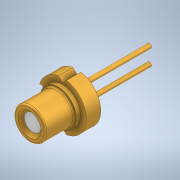
# Autodesk Inventor part: CAN_φ3.3
Saved by Autodesk Inventor 2020 (Build 240168000, 168)
## iProperties
Created: 2020-03-16
Part Number: CAN_φ3.3
Material: 黄铜，软黄
Document SubType Name: Modeling
Designer: John
Mass: 0.447561 g
Surface Area: 1.18166 cm^2
Volume: 0.0528407 cm^3
Density: 8.47 g/cm^3
Appearance: 黄铜 - 缎光
Author: John
Autodesk Inventor part; units mm, degrees
ref_plane "YZ Plane" through (0, 0, 0) normal (1, 0, 0) x (0, 1, 0)
ref_plane "XZ Plane" through (0, 0, 0) normal (0, 1, 0) x (-1, 0, 0)
ref_plane "XY Plane" through (0, 0, 0) normal (0, 0, 1) x (1, 0, 0)
sketch "草图1" plane through (0, 0, 0) normal (0, 0, 1) x (1, 0, 0)
  circle A0 centre (0, 0) radius 1.65
  circle A1 centre (0, 0) radius 0.55 construction
  line L0 (0, 1.65) -> (0, 1.35)
  line L1 (0, 1.35) -> (0.2766, 1.6266)
  line L2 (0, 1.35) -> (-0.2766, 1.6266)
  line L3 (0, 1.35) -> (0.3912, 1.35) construction
  line L4 (0, 0) -> (0, 1.65) construction
  line L5 (0, 0) -> (-1.65, 0) construction
  line L6 (0, 0) -> (0, -1.65) construction
  circle A2 centre (0, 0.55) radius 0.15
  circle A3 centre (0, -0.55) radius 0.15
  circle A4 centre (-0.55, 0) radius 0.15
  circle A5 centre (-0.55, 0) radius 0.4
  line L7 (0, -1.65) -> (0, -1.35)
  line L8 (0, -1.35) -> (0.2766, -1.6266)
  line L9 (0, -1.35) -> (-0.2766, -1.6266)
  line L10 (0, -1.35) -> (0.3912, -1.35) construction
  line L11 (-1.35, 0) -> (-1.35, 0.5)
  line L12 (-1.35, 0.5) -> (-1.5724, 0.5)
  line L13 (-1.35, 0) -> (-1.35, -0.5)
  line L14 (-1.35, -0.5) -> (-1.5724, -0.5)
  point P0 (-0.2766, -1.6266)
  point P1 (0.2766, -1.6266)
  dimension "d0" = 3.3
  dimension "d1" = 1.1
  dimension "d5" = 0.3
  dimension "d6" = 45
  dimension "d7" = 135
  dimension "d8" = 0.3
  dimension "d9" = 0.3
  dimension "d10" = 0.3
  dimension "d11" = 0.8
  dimension "d12" = 0.5
  dimension "d13" = 0.5
  dimension "d14" = 0.3
  constraints: 30 end point, 6 symmetric about line, 5 centre point, 5 point on line, 3 coincident, 3 perpendicular, 3 point on circle, 3 vertical, 2 horizontal, 1 collinear, 1 equal length, 10 other
  measures "d1" diameter of A1
  measures "d5" distance of L0.start L0.end
  measures "d6" angle of L1 L0
  measures "d7" angle of L3 L2
  measures "d8" diameter of A2
  measures "d9" diameter of A3
  measures "d10" diameter of A4
  measures "d11" diameter of A5
  measures "d12" distance of L11.start L11.end
  measures "d13" distance of L11.start L13.end
  measures "d14" distance of L11.start L5.end
extrude "拉伸1" add sketch "草图1" along normal blind 1 contours A0 L8 L9 L14 L13 L11 L12 L2 L1 | A2 | A3 | A4 | A5
extrude "拉伸2" add sketch "草图1" against normal blind 5 contours A2 | A3 | A4
extrude "拉伸3" add sketch "草图1" against normal blind 0.3 contours A5
sketch "草图2" plane through (0, 0, 1) normal (0, 0, 1) x (1, 0, 0)
  circle A0 centre (0, 0) radius 1.1
  circle A1 centre (0, 0) radius 1.25
  dimension "d21" = 2.2
  dimension "d22" = 2.5
  constraints: 2 centre point, 2 coincident
  measures "d21" diameter of A0
  measures "d22" diameter of A1
extrude "拉伸4" add sketch "草图2" along normal blind 2.27 contours A0
extrude "拉伸5" add sketch "草图2" along normal blind 0.3
sketch "草图3" plane through (0, 0, 0) normal (1, 0, 0) x (0, 1, 0)
  line L0 (1.1, 3.27) -> (-1.1, 3.27) projected
  line L1 (0, 3.27) -> (-0.8, 3.27)
  line L2 (-0.8, 3.27) -> (-0.5879, 3.0579)
  line L3 (-0.5879, 3.0579) -> (0, 3.0579)
  line L4 (0, 3.0579) -> (0, 3.27)
  point P0 (0, 0)
  dimension "d27" = 0.8
  dimension "d28" = 0.3
  dimension "d29" = 45
  constraints: 8 end point, 1 midpoint, 1 parallel, 1 perpendicular, 1 point on line
  measures "d27" distance of L1.start L1.end
  measures "d28" distance of L1.end L2.end
  measures "d29" angle of L2 L1
revolve "旋转1" cut sketch "草图3" angle 360 about axis through (0, 0, 3.0579) along (0, 0, 1)
fillet "圆角1" radius 0.1 2 edges at (-1.1, 0, 3.27) (-1.1, 0, 1.3)
